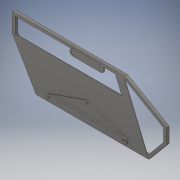
# Autodesk Inventor part: Cabin Wall
Saved by Autodesk Inventor 2019 (Build 230136000, 136)
## iProperties
Created: 2019-08-25
Part Number: Cabin Wall
Material: Steel, Mild
Document SubType Name: Modeling
Designer: DIBYOJYOTI
Density: 7.85 g/cm^3
Appearance: Semi-Polished
Mass: 481.734 g
Surface Area: 649.084 cm^2
Volume: 61.3673 cm^3
Author: DIBYOJYOTI
Autodesk Inventor part; units mm, degrees
ref_plane "YZ Plane" through (0, 0, 0) normal (1, 0, 0) x (0, 1, 0)
ref_plane "XZ Plane" through (0, 0, 0) normal (0, 1, 0) x (-1, 0, 0)
ref_plane "XY Plane" through (0, 0, 0) normal (0, 0, 1) x (1, 0, 0)
sketch "Sketch2" plane through (0, 0, 0) normal (0, 0, 1) x (1, 0, 0)
  circle A0 centre (50, 110) radius 3
  circle A1 centre (0, 0) radius 3
  circle A2 centre (160, 0) radius 3
  circle A3 centre (80, 30) radius 2.05
  circle A4 centre (110, 110) radius 3
  line L0 (50, 110) -> (110, 110) construction
  line L1 (50, 103) -> (110, 103)
  line L2 (110, 117) -> (50, 117)
  arc A5 (50, 117) -> (50, 103) centre (50, 110) ccw
  arc A6 (110, 103) -> (110, 117) centre (110, 110) ccw
  line L3 (160, 0) -> (157, 0) construction
  line L4 (3, 0) -> (0, 0) construction
  line L5 (0, 0) -> (160, 0) construction
  line L6 (0, -7) -> (160, -7)
  line L7 (160, 7) -> (0, 7)
  arc A7 (0, 7) -> (0, -7) centre (0, 0) ccw
  arc A8 (160, -7) -> (160, 7) centre (160, 0) ccw
  arc A9 (81.6455, 34.7215) -> (78.3545, 34.7215) centre (80, 30) ccw
  line L8 (-2.3038, 6.61) -> (78.3545, 34.7215)
  line L9 (162.3038, 6.61) -> (81.6455, 34.7215)
  point P0 (80, 110)
  point P1 (80, 0)
  dimension "d1" = 6
  dimension "d2" = 6
  dimension "d0" = 6
  dimension "d3" = 4.1
  dimension "d5" = 6
  dimension "d11" = 80
  dimension "d12" = 14
  dimension "d13" = 10
  dimension "d20" = 160
  dimension "d21" = 110
  dimension "d22" = 60
  dimension "d23" = 30
  constraints: 24 end point, 12 point on circle, 12 tangent, 8 centre point, 4 coincident, 3 horizontal, 2 horizontal alignment, 2 midpoint, 2 parallel, 1 collinear, 4 other
  measures "d0" diameter of A0
  measures "d3" diameter of A3
  measures "d5" diameter of A4
  measures "d11" horizontal distance of A3.centre point (0, 0)
  measures "d12" diameter of A8
  measures "d13" diameter of A9
  measures "d20" distance of point (0, 0) L3.start
  measures "d21" vertical distance of point (0, 0) A0.centre
  measures "d22" distance of A0.centre L0.end
  measures "d23" vertical distance of point (0, 0) A3.centre
extrude "Extrusion1" add sketch "Sketch2" against normal blind 1
extrude "Extrusion2" add sketch "Sketch2" along normal blind 2 contours A7 L7 A8 L6
extrude "Extrusion3" add sketch "Sketch2" along normal blind 1 contours A5 L2 A6 L1
sketch3d "3D Sketch1"
ref_plane "Work Plane1" through (110, 117, -4) normal (0, 0, -1) x (-1, 0, 0)
sketch "Sketch3" plane through (110, 117, -4) normal (0, 0, -1) x (-1, 0, 0)
  line L0 (0, 0) -> (-50, 0)
  line L1 (0, 0) -> (50, 0) construction
  line L2 (-50, 0) -> (-136.6025, -50)
  line L3 (-50, 0) -> (50, 0) construction
  line L4 (-136.6025, -50) -> (-136.6025, -80)
  line L5 (-50, -124) -> (110, -124) projected
  line L6 (-50, -124) -> (-100, -124)
  line L7 (-100, -124) -> (-136.6025, -80)
  line L8 (110, -124) -> (140, -124)
  line L9 (140, -124) -> (190, -37.3975)
  line L10 (60, 0) -> (0, 0) projected
  line L11 (0, 0) -> (60, 0)
  line L12 (60, 0) -> (190, 0)
  line L13 (190, 0) -> (190, -37.3975)
  point P0 (110, -117)
  dimension "d25" = 50
  dimension "d26" = 180
  dimension "d27" = 100
  dimension "d28" = 150
  dimension "d29" = 30
  dimension "d30" = 50
  dimension "d31" = 30
  dimension "d32" = 100
  dimension "d33" = 120
  dimension "d34" = 190
  dimension "d35" = 37.3975
  constraints: 24 end point, 5 horizontal, 2 equal length, 1 collinear, 1 perpendicular, 1 point on line, 1 vertical
  measures "d25" distance of L0.start L0.end
  measures "d26" angle of L0 L1
  measures "d27" distance of L0.end L2.end
  measures "d28" angle of L2 L3
  measures "d29" distance of L2.end L4.end
  measures "d30" distance of L5.start L6.end
  measures "d31" distance of L5.end L8.end
  measures "d32" distance of L8.end L9.end
  measures "d33" angle of L9 L8
  measures "d34" distance of L12.end L0.start
  measures "d35" distance of L12.end L9.end
ref_plane "Work Plane2" through (-80, 117, -4) normal (-1, 0, 0) x (0, -1, 0)
sketch "Sketch4" plane through (-80, 117, -4) normal (-1, 0, 0) x (0, -1, 0)
  line L0 (3, 3) -> (-3, 3)
  line L1 (-3, 3) -> (-3, -3)
  line L2 (-3, -3) -> (3, -3)
  line L3 (3, -3) -> (3, 3)
  line L4 (3, 3) -> (-3, -3) construction
  line L5 (-3, 3) -> (3, -3) construction
  point P0 (117, 4)
  point P1 (0, 0)
  dimension "d36" = 6
  dimension "d37" = 6
  constraints: 12 end point, 2 midpoint, 2 parallel, 1 horizontal, 1 perpendicular
  measures "d36" distance of L2.end L1.end
  measures "d37" distance of L1.end L0.end
sweep "Sweep1" add profiles "Sketch4" path "Sketch3" path curves L12 L11 L0 L2 L4 L7 L6 L5 L8 L9 L13
ref_plane "Work Plane3" through (249.6025, 52.3237, -1) normal (0, 0, 1) x (1, 0, 0)
sketch "Sketch5" plane through (249.6025, 52.3237, -1) normal (0, 0, 1) x (1, 0, 0)
  line L0 (-41.0092, -56.3237) -> (-277.8705, -56.3237) projected
  line L1 (-90.4064, 61.6763) -> (-41.0092, -56.3237)
  line L2 (-41.0092, -56.3237) -> (-277.8705, -56.3237)
  line L3 (-277.8705, -56.3237) -> (-326.6025, 28.0827) projected
  line L4 (-277.8705, -56.3237) -> (-326.6025, 28.0827)
  line L5 (-326.6025, 28.0827) -> (-326.6025, 61.6763) projected
  line L6 (-326.6025, 28.0827) -> (-326.6025, 61.6763)
  line L7 (-326.6025, 61.6763) -> (-90.4064, 61.6763)
  line L8 (-76.3434, 28.0827) -> (-96.3434, 28.0827)
  line L9 (-96.3434, 28.0827) -> (-110.4064, 61.6763)
  line L10 (-326.6025, 61.6763) -> (-90.4064, 61.6763) projected
  line L11 (-326.6025, 28.0827) -> (-326.6025, 61.6763) projected
  line L12 (-326.6025, 61.6763) -> (-205.3471, 61.6763) projected
  line L13 (-326.6025, 28.0827) -> (-279.094, 28.0827) construction
  line L14 (-293.0089, 61.6763) -> (-110.4064, 61.6763)
  line L15 (-133.858, 61.6763) -> (-90.4064, 61.6763) projected
  line L16 (-326.6025, 28.0827) -> (-96.3434, 28.0827)
  point P0 (-249.6025, -52.3237)
  dimension "d44" = 20
  constraints: 20 end point, 4 collinear, 3 point on line, 2 perpendicular, 1 horizontal, 1 parallel
  measures "d44" distance of L8.start L8.end
extrude "Extrusion5" add sketch "Sketch5" against normal blind 1
extrude "Extrusion6" cut sketch "Sketch5" against normal blind 1 contours L5 L7 L9 L16
body "Solid1"
